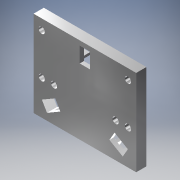
# Autodesk Inventor part: trackball_base
Saved by Autodesk Inventor 2018 (Build 220112000, 112)
## iProperties
Created: 2018-04-03
Part Number: trackball_base
Material: アルミニウム 6061
Document SubType Name: Modeling
Designer: NaMACHAN
Density: 2.7 g/cm^3
Appearance: アルミニウム - フラット
Author: NaMACHAN
Autodesk Inventor part; units mm, degrees
ref_plane "YZ Plane" through (0, 0, 0) normal (1, 0, 0) x (0, 1, 0)
ref_plane "XZ Plane" through (0, 0, 0) normal (0, 1, 0) x (-1, 0, 0)
ref_plane "XY Plane" through (0, 0, 0) normal (0, 0, 1) x (1, 0, 0)
sketch "スケッチ1" plane through (0, 0, 0) normal (0, 1, 0) x (-1, 0, 0)
  line L0 (-25, -16.9) -> (25, -16.9)
  line L1 (25, -16.9) -> (25, 25)
  line L2 (25, 25) -> (-25, 25)
  line L3 (-25, 25) -> (-25, -16.9)
  point P0 (0, 0)
  point P1 (0, 25)
  dimension "d0" = 50
  dimension "d62" = 25
  dimension "d63" = 16.9
  constraints: 8 end point, 2 parallel, 1 horizontal, 1 midpoint, 1 perpendicular, 1 vertical alignment
  measures "d0" distance of L2.end L1.end
  measures "d62" distance from line of L2 point (0, 0)
  measures "d63" distance from line of L0 point (0, 0)
extrude "押し出し1" add sketch "スケッチ1" along normal blind 5
sketch "スケッチ2" plane through (0, 5, 0) normal (0, 1, 0) x (1, 0, 0)
  circle A0 centre (0, 0) radius 16.5
  dimension "d4" = 33
  constraints: 1 centre point, 1 coincident
  measures "d4" diameter of A0
extrude "押し出し2" cut sketch "スケッチ2" against normal blind 5
sketch "スケッチ3" plane through (0, 5, 0) normal (0, 1, 0) x (1, 0, 0)
  line L0 (-6, -17.5) -> (6, -17.5)
  line L1 (6, -17.5) -> (6, -20.5)
  line L2 (6, -20.5) -> (-6, -20.5)
  line L3 (-6, -20.5) -> (-6, -17.5)
  line L4 (-6, -17.5) -> (6, -20.5) construction
  line L5 (6, -17.5) -> (-6, -20.5) construction
  line L6 (-14.7535, 15.4462) -> (-20.7535, 5.0538)
  line L7 (-20.7535, 5.0538) -> (-18.1554, 3.5538)
  line L8 (-18.1554, 3.5538) -> (-12.1554, 13.9462)
  line L9 (-12.1554, 13.9462) -> (-14.7535, 15.4462)
  line L10 (-14.7535, 15.4462) -> (-18.1554, 3.5538) construction
  line L11 (-20.7535, 5.0538) -> (-12.1554, 13.9462) construction
  line L12 (-25, 16.9) -> (-25, -25) projected
  line L13 (12.1554, 13.9462) -> (18.1554, 3.5538)
  line L14 (18.1554, 3.5538) -> (20.7535, 5.0538)
  line L15 (20.7535, 5.0538) -> (14.7535, 15.4462)
  line L16 (14.7535, 15.4462) -> (12.1554, 13.9462)
  line L17 (12.1554, 13.9462) -> (20.7535, 5.0538) construction
  line L18 (18.1554, 3.5538) -> (14.7535, 15.4462) construction
  line L19 (25, -25) -> (25, 16.9) projected
  point P0 (0, 0)
  point P1 (0, -19)
  point P2 (-16.4545, 9.5)
  point P3 (16.4545, 9.5)
  point P4 (16.4545, 9.5)
  point P5 (16.4545, 9.5)
  dimension "d7" = 120
  dimension "d8" = 120
  dimension "d9" = 19
  dimension "d10" = 19
  dimension "d11" = 19
  dimension "d12" = 3
  dimension "d13" = 12
  dimension "d14" = 30
  dimension "d15" = 12
  dimension "d16" = 3
  dimension "d17" = 30
  dimension "d18" = 3
  dimension "d19" = 12
  constraints: 36 end point, 7 midpoint, 6 parallel, 3 perpendicular, 1 coincident, 1 horizontal, 1 vertical alignment
  measures "d9" distance of point (0, 0) point (0, -19)
  measures "d10" distance of point (-16.454, 9.5) point (0, 0)
  measures "d11" distance of point (16.454, 9.5) point (0, 0)
  measures "d12" distance of L0.end L1.end
  measures "d13" distance between parallel lines of L1 L3
  measures "d14" angle of L12 L6
  measures "d15" distance of L7.end L8.end
  measures "d16" distance of L6.end L7.end
  measures "d17" angle of L19 L15
  measures "d18" distance of L15.end L13.start
  measures "d19" distance of L13.start L13.end
extrude "押し出し3" cut sketch "スケッチ3" against normal blind 3
sketch "スケッチ4" plane through (0, 5, 0) normal (0, 1, 0) x (1, 0, 0)
  line L0 (2.5, -15.25) -> (2.5, -22.75)
  line L1 (2.5, -22.75) -> (-2.5, -22.75)
  line L2 (-2.5, -22.75) -> (-2.5, -15.25)
  line L3 (-2.5, -15.25) -> (2.5, -15.25)
  line L4 (2.5, -15.25) -> (-2.5, -22.75) construction
  line L5 (2.5, -22.75) -> (-2.5, -15.25) construction
  line L6 (18.4521, 13.5401) -> (11.9569, 9.7901)
  line L7 (11.9569, 9.7901) -> (14.4569, 5.4599)
  line L8 (14.4569, 5.4599) -> (20.9521, 9.2099)
  line L9 (20.9521, 9.2099) -> (18.4521, 13.5401)
  line L10 (18.4521, 13.5401) -> (14.4569, 5.4599) construction
  line L11 (11.9569, 9.7901) -> (20.9521, 9.2099) construction
  line L12 (25, -25) -> (25, 16.9) projected
  line L13 (-18.4521, 13.5401) -> (-11.9569, 9.7901)
  line L14 (-11.9569, 9.7901) -> (-14.4569, 5.4599)
  line L15 (-14.4569, 5.4599) -> (-20.9521, 9.2099)
  line L16 (-20.9521, 9.2099) -> (-18.4521, 13.5401)
  line L17 (-18.4521, 13.5401) -> (-14.4569, 5.4599) construction
  line L18 (-11.9569, 9.7901) -> (-20.9521, 9.2099) construction
  line L19 (-25, 16.9) -> (-25, -25) projected
  point P0 (0, 0)
  point P1 (16.4545, 9.5)
  point P2 (0, -19)
  point P3 (-16.4545, 9.5)
  dimension "d28" = 120
  dimension "d29" = 120
  dimension "d30" = 19
  dimension "d31" = 19
  dimension "d32" = 19
  dimension "d33" = 30
  dimension "d34" = 7.5
  dimension "d35" = 5
  dimension "d38" = 7.5
  dimension "d39" = 5
  dimension "d40" = 5
  dimension "d41" = 7.5
  dimension "d42" = 30
  constraints: 36 end point, 6 midpoint, 6 parallel, 3 perpendicular, 1 vertical, 1 vertical alignment
  measures "d30" distance of point (0, 0) point (0, -19)
  measures "d31" distance of point (-16.454, 9.5) point (0, 0)
  measures "d32" distance of point (16.454, 9.5) point (0, 0)
  measures "d33" angle of L12 L9
  measures "d34" distance of L6.start L6.end
  measures "d35" distance of L6.end L7.end
  measures "d38" distance of L1.end L2.end
  measures "d39" distance of L2.end L0.start
  measures "d40" distance of L15.end L13.start
  measures "d41" distance of L14.end L15.end
  measures "d42" angle of L19 L16
extrude "押し出し4" cut sketch "スケッチ4" against normal blind 5
sketch "スケッチ5" plane through (0, 5, 0) normal (0, 1, 0) x (1, 0, 0)
  line L0 (-25, -25) -> (25, -25) projected
  line L1 (25, 16.9) -> (-25, 16.9) projected
  line L2 (-25, 16.9) -> (-25, -25) projected
  line L3 (25, -25) -> (25, 16.9) projected
  point P0 (0, 0)
  point P1 (21, -20)
  point P2 (-21, -20)
  point P3 (-21, 0)
  point P4 (21, 0)
  point P5 (15, 0)
  point P6 (-15, 0)
  dimension "d45" = 5
  dimension "d48" = 5
  dimension "d49" = 4
  dimension "d50" = 4
  dimension "d51" = 4
  dimension "d52" = 4
  dimension "d60" = 6
  dimension "d61" = 6
  dimension "d64" = 20
  constraints: 3 horizontal alignment
  measures "d45" distance from line of L0 point (21, -20)
  measures "d48" distance from line of L0 point (-21, -20)
  measures "d49" distance from line of L2 point (-21, -20)
  measures "d50" distance from line of point (-21, 0) L2
  measures "d51" distance from line of L3 point (21, 0)
  measures "d52" distance from line of L3 point (21, -20)
  measures "d60" distance of point (-21, 0) point (-15, 0)
  measures "d61" distance of point (21, 0) point (15, 0)
  measures "d64" distance of point (21, 0) point (21, -20)
hole "穴1" at (21, 5, 20) at (-21, 5, 20) at (-21, 5, 0) at (21, 5, 0) at (15, 5, 0) at (-15, 5, 0) direction (0, -1, 0) diameter 3 end through all
